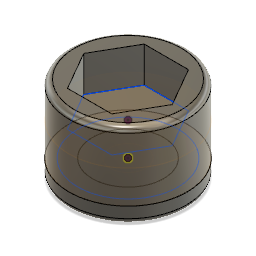
Connector_Plunger_only (Autodesk Fusion 360 design; units mm, degrees)
Autodesk Fusion 360 part; units mm, degrees
sketch "Sketch4" plane through (0, 11.5, 0) normal (0, 1, 0) x (-1, 0, 0) in component "Plunger"
  circle A0 centre (0, 0) radius 3.25
  circle A1 centre (0, 0) radius 6.5
  circle A2 centre (0, 0) radius 10.75
  dimension "d20" = 13
  dimension "d21" = 21.5
  measures "d20" diameter of A1
  measures "d21" diameter of A2
extrude "Extrude3" add sketch "Sketch4" against normal blind 3 contours A2 in component "Plunger"
sketch "Sketch5" plane through (0, 11.5, 0) normal (0, 1, 0) x (-1, 0, 0) in component "Plunger"
  circle A0 centre (0, 0) radius 6.5
  circle A1 centre (0, 0) radius 10.75
  circle A2 centre (0, 0) radius 9.15
extrude "Extrude4" add sketch "Sketch5" along normal blind 6 contours A0 | A1 | A2 in component "Plunger"
sketch "Sketch1" plane through (0, 11.5, 0) normal (0, -1, 0) x (1, 0, 0)
  circle A0 centre (0, 0) radius 6.5
  circle A1 centre (0, 0) radius 3.25
  dimension "d29" = 6.5
  measures "d29" diameter of A1
extrude "Extrude6" cut sketch "Sketch1" against normal blind 3.5 contours A1 in component "Plunger"
sketch "Sketch7" plane through (0, 17.5, 0) normal (0, 1, 0) x (-1, 0, 0) in component "Plunger"
  circle A0 centre (0, 0) radius 10.75
  line L0 (4.0415, -7) -> (8.0829, 0)
  line L1 (8.0829, 0) -> (4.0415, 7)
  line L2 (4.0415, 7) -> (-4.0415, 7)
  line L3 (-4.0415, 7) -> (-8.0829, 0)
  line L4 (-8.0829, 0) -> (-4.0415, -7)
  line L5 (-4.0415, -7) -> (4.0415, -7)
  dimension "d32" = 7
  measures "d32" distance of A0.centre L5
extrude "Extrude7" add sketch "Sketch7" along normal blind 6.5 in component "Plunger"
fillet "Fillet1" radius 1 1 edges at (6.0601, 8.5, -2.3505) in component "Plunger"
fillet "Fillet2" radius 1 1 edges at (10.0225, 8.5, 3.8874) in component "Plunger"
fillet "Fillet3" radius 1 1 edges at (10.0225, 24, -3.8874) in component "Plunger"
component "Plunger" placed x (1, 0, 0) y (0, 1, 0) z (0, 0, 1) at (0, 0, 0)
